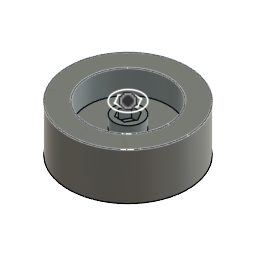
wheel_85mm_v0_1 (Autodesk Fusion 360 design; units mm, degrees)
part number: 2026-05-27-21-11-46-557
Autodesk Fusion 360 part; units mm, degrees
sketch "草图1" plane through (0, 0, 0) normal (0, 1, 0) x (1, 0, 0)
  circle A0 centre (0, 0) radius 42.5
  circle A1 centre (0, 0) radius 28.8
  circle A2 centre (0, 0) radius 10
  line L0 (-3.4641, 6) -> (3.4641, 6)
  line L1 (3.4641, 6) -> (6.9282, 0)
  line L2 (6.9282, 0) -> (3.4641, -6)
  line L3 (3.4641, -6) -> (-3.4641, -6)
  line L4 (-3.4641, -6) -> (-6.9282, 0)
  line L5 (-6.9282, 0) -> (-3.4641, 6)
  line L6 (0, 6) -> (0, -6) construction
  dimension "d1" = 85
  dimension "d2" = 57.6
  dimension "d3" = 20
  dimension "d11" = 120
  dimension "d12" = 120
  dimension "d13" = 12
  constraint coincident A0.centre A1.centre
  constraint concentric A0 A1
  constraint concentric A1 A2
  constraint horizontal L0
  constraint parallel L0 L3
  constraint equal L0 L1
  constraint equal L0 L2
  constraint equal L0 L3
  constraint equal L0 L4
  constraint equal L0 L5
  constraint coincident L0 L6.start
  constraint coincident L3 L6.end
  constraint perpendicular L3 L6
  constraint midpoint L6 A0.centre
  constraint symmetric L1 L5 L6
  measures "d1" diameter of A0
  measures "d2" diameter of A1
  measures "d3" diameter of A2
  measures "d11" angle of L4 L5
  measures "d12" angle of L0 L1
  measures "d13" distance of L0 L3
extrude "拉伸1" add sketch "草图1" against normal blind 33.4 contours A0 | A1 | A2 | L0 L1 L2 L3 L4 L5
extrude "拉伸2" cut sketch "草图1" against normal blind 17 contours A1
extrude "拉伸3" cut sketch "草图1" against normal blind 8.3 contours A2 | L0 L1 L2 L3 L4 L5
extrude "拉伸4" cut sketch "草图1" against normal blind 15.3 contours L0 L1 L2 L3 L4 L5
equation "d14 = -7 mm - 8.3 mm"
